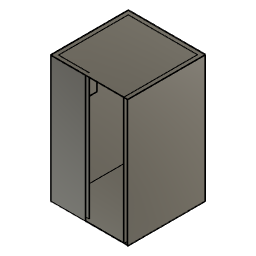
photo-booth v3 (Autodesk Fusion 360 design; units mm, degrees)
Autodesk Fusion 360 part; units mm, degrees
note: some values were not read from the file. Set by a fixed rule: which face or edge a step refers to.
sketch "Sketch1" plane through (0, 0, 0) normal (0, 0, 1) x (1, 0, 0)
  line L0 (0, 0) -> (1200, 0)
  line L1 (1200, 0) -> (1200, 1210)
  line L2 (1200, 1210) -> (0, 1210)
  line L3 (0, 1210) -> (0, 0)
  dimension "d1" = 1200
  dimension "d2" = 1210
  constraint horizontal L0
  constraint vertical L1
  constraint horizontal L2
  constraint vertical L3
  constraint coincident L0.start L3.end
  measures "d1" distance of L0.start L0.end
  measures "d2" distance of L0.start L2.end
extrude "Extrude1" add sketch "Sketch1" along normal blind 9 makes body 1 in component "Component"
sketch "Sketch2" plane through (1200, 0, 0) normal (1, 0, 0) x (0, 1, 0)
  line L0 (0, 0) -> (1210, 0)
  line L1 (1210, 0) -> (1210, 9)
  line L2 (1210, 9) -> (0, 9)
  line L3 (0, 9) -> (0, 0)
  line L4 (-9, 0) -> (1209, 0)
  line L5 (1209, 0) -> (1209, 2000)
  line L6 (1209, 2000) -> (-9, 2000)
  line L7 (-9, 2000) -> (-9, 0)
  dimension "d5" = 1218
  dimension "d6" = 2000
  constraint horizontal L4
  constraint vertical L5
  constraint horizontal L6
  constraint vertical L7
  measures "d5" distance of L4.start L4.end
  measures "d6" distance of L4.start L6.end
extrude "Extrude2" add sketch "Sketch2" along normal blind 9 bodies 1 in component "Component"
sketch "Sketch3" plane through (0, 1210, 0) normal (0, 1, 0) x (-1, 0, 0)
  line L0 (-1209, 0) -> (0, 0)
  line L1 (0, 0) -> (0, 9)
  line L2 (0, 9) -> (-1209, 9)
  line L3 (-1209, 0) -> (10, 0)
  line L4 (10, 0) -> (10, 2000)
  line L5 (10, 2000) -> (-1209, 2000)
  line L6 (-1209, 2000) -> (-1209, 0)
  line L7 (-1209, 9) -> (-1209, 0)
  dimension "d9" = 1219
  dimension "d10" = 2000
  constraint horizontal L3
  constraint vertical L4
  constraint horizontal L5
  constraint vertical L6
  constraint coincident L0.start L3.start
  measures "d9" distance of L0.start L3.end
  measures "d10" distance of L0.start L5.end
extrude "Extrude3" add sketch "Sketch3" along normal blind 9 separate body makes body 2 in component "Component"
sketch "Sketch6" plane through (0, 0, 0) normal (-1, 0, 0) x (0, -1, 0)
  line L0 (-1210, 0) -> (0, 0)
  line L1 (0, 0) -> (0, 9)
  line L2 (0, 9) -> (-1210, 9)
  line L3 (-1210, 9) -> (-1210, 0)
  line L4 (-1210, 0) -> (8, 0)
  line L5 (8, 0) -> (8, 2000)
  line L6 (8, 2000) -> (-1210, 2000)
  line L7 (-1210, 2000) -> (-1210, 0)
  dimension "d19" = 1218
  dimension "d20" = 2000
  constraint horizontal L4
  constraint vertical L5
  constraint horizontal L6
  constraint vertical L7
  measures "d19" distance of L0.start L4.end
  measures "d20" distance of L0.start L6.end
extrude "Extrude1'" add sketch "Sketch6" along normal blind 9 separate body makes body 3 in component "Component'"
sketch "Sketch7" plane through (1200, 0, 0) normal (-1, 0, 0) x (0, -1, 0)
  line L0 (0, 9) -> (0, 0)
  line L1 (0, 0) -> (9, 0)
  line L2 (9, 0) -> (9, 2000)
  line L3 (9, 2000) -> (-1209, 2000)
  line L4 (-1209, 2000) -> (-1209, 9)
  line L5 (-1209, 9) -> (0, 9)
  line L6 (-1209, 9) -> (-1159, 9)
  line L7 (-1159, 9) -> (-1159, 2000)
  line L8 (-1159, 2000) -> (-1209, 2000)
  line L9 (-1209, 2000) -> (-1209, 9)
  dimension "d23" = 50
  constraint horizontal L6
  constraint vertical L7
  constraint horizontal L8
  constraint vertical L9
  constraint coincident L4.end L5.start
  measures "d23" distance of L4.end L6.end
extrude "Extrude1''" add sketch "Sketch7" along normal blind 50 separate body contours L3 L4 L5 L6 L7 L8 L9 makes body 4
sketch "Sketch8" plane through (0, 0, 9) normal (0, 0, 1) x (-1, 0, 0)
  line L0 (0, -1210) -> (0, 0)
  line L1 (0, 0) -> (-1200, 0)
  line L2 (-1200, 0) -> (-1200, -1209)
  line L3 (-1209, -1210) -> (0, -1210)
  line L4 (0, -1210) -> (-50, -1210)
  line L5 (-50, -1210) -> (-50, -1160)
  line L6 (-50, -1160) -> (0, -1160)
  line L7 (0, -1160) -> (0, -1210)
  line L8 (-1200, -1209) -> (-1209, -1209)
  line L9 (-1209, -1209) -> (-1209, -1210)
  constraint horizontal L4
  constraint vertical L5
  constraint horizontal L6
  constraint vertical L7
  constraint coincident L0.start L3.end
extrude "Extrude2'" add sketch "Sketch8" along normal blind 1991 separate body contours L0 L3 L4 L5 L6 L7 makes body 5
sketch "Sketch9" plane through (0, 0, 9) normal (0, 0, 1) x (-1, 0, 0)
  line L0 (0, -1210) -> (0, 0)
  line L1 (0, 0) -> (-1200, 0)
  line L2 (-1200, 0) -> (-1200, -1209)
  line L3 (-1209, -1210) -> (0, -1210)
  line L4 (0, 0) -> (-50, 0)
  line L5 (-50, 0) -> (-50, -50)
  line L6 (-50, -50) -> (0, -50)
  line L7 (0, -50) -> (0, 0)
  line L8 (-1200, -1209) -> (-1209, -1209)
  line L9 (-1209, -1209) -> (-1209, -1210)
  constraint horizontal L4
  constraint vertical L5
  constraint horizontal L6
  constraint vertical L7
  constraint coincident L0.end L1.start
extrude "Extrude3'" add sketch "Sketch9" along normal blind 1991 separate body contours L0 L1 L4 L5 L6 L7 makes body 6
sketch "Sketch10" plane through (0, 1160, 0) normal (0, -1, 0) x (1, 0, 0)
  line L0 (0, 9) -> (50, 9)
  line L1 (50, 9) -> (50, 2000)
  line L2 (50, 2000) -> (0, 2000)
  line L3 (0, 2000) -> (0, 9)
  line L4 (0, 9) -> (50, 9)
  line L5 (50, 9) -> (50, 59)
  line L6 (50, 59) -> (0, 59)
  line L7 (0, 59) -> (0, 9)
  dimension "d30" = 50
  constraint horizontal L4
  constraint vertical L5
  constraint horizontal L6
  constraint vertical L7
  constraint coincident L0.start L3.end
  measures "d30" distance of L0.start L6.end
extrude "Extrude4" add sketch "Sketch10" along normal blind 1100 separate body contours L0 L1 L3 L4 L5 L6 L7 makes body 7
sketch "Sketch11" plane through (0, 1160, 0) normal (0, -1, 0) x (1, 0, 0)
  line L0 (0, 9) -> (50, 9)
  line L1 (50, 9) -> (50, 2000)
  line L2 (50, 2000) -> (0, 2000)
  line L3 (0, 2000) -> (0, 9)
  line L4 (0, 2000) -> (50, 2000)
  line L5 (50, 2000) -> (50, 1950)
  line L6 (50, 1950) -> (0, 1950)
  line L7 (0, 1950) -> (0, 2000)
  constraint horizontal L4
  constraint vertical L5
  constraint horizontal L6
  constraint vertical L7
  constraint coincident L1 L5.end
  constraint coincident L2.end L3.start
extrude "Extrude5" add sketch "Sketch11" along normal blind 1100 separate body contours L1 L2 L3 L4 L5 L6 L7 makes body 8
sketch "Sketch12" plane through (0, 0, 0) normal (1, 0, 0) x (0, 1, 0)
  line L0 (1210, 0) -> (1210, 2000)
  line L1 (1210, 2000) -> (-8, 2000)
  line L2 (-8, 2000) -> (-8, 0)
  line L3 (-8, 0) -> (1210, 0)
  line L4 (708, -17) -> (708, 1123) construction
  line L5 (600.0031, 1126.4153) -> (50.0031, 1126.4153) construction
  line L6 (525, 975) -> (710, 975)
  line L7 (710, 975) -> (710, 1310)
  line L8 (710, 1310) -> (525, 1310)
  line L9 (525, 1310) -> (525, 975)
  line L10 (525, 2000) -> (475, 2000)
  line L11 (475, 2000) -> (475, 50)
  line L12 (475, 50) -> (525, 50)
  line L13 (525, 50) -> (525, 2000)
  line L14 (710, 60) -> (660, 60)
  line L15 (660, 60) -> (660, 1950.3478)
  line L16 (660, 1950.3478) -> (710, 1950.3478)
  line L17 (710, 1950.3478) -> (710, 60)
  line L18 (525, 1950.1089) -> (475, 1950.1089)
  dimension "d35" = 1140
  dimension "d36" = 550
  dimension "d37" = 50
  dimension "d38" = 50
  constraint perpendicular L3 L4
  constraint parallel L1 L5
  constraint horizontal L6
  constraint vertical L7
  constraint horizontal L8
  constraint vertical L9
  constraint horizontal L10
  constraint vertical L11
  constraint horizontal L12
  constraint vertical L13
  constraint coincident L1 L10.start
  constraint horizontal L14
  constraint vertical L15
  constraint horizontal L16
  constraint vertical L17
  constraint coincident L13 L18.start
  constraint coincident L11 L18.end
  constraint perpendicular L11 L18
  measures "d35" distance of L4.start L4.end
  measures "d36" distance of L5.start L5.end
  measures "d37" distance of L10.start L10.end
  measures "d38" distance of L14.start L14.end
extrude "Extrude6" add sketch "Sketch12" along normal blind 50 separate body contours L9 L11 L12 L13 L18 | L8 L15 L16 L17 | L6 L7 L8 L15 L17 | L6 L14 L15 L17 makes body 9 at (16.6667, 525, 683.3696) makes body 10 at (0, 676.6667, 1320.2319)
sketch "Sketch13" plane through (0, 0, 0) normal (1, 0, 0) x (0, 1, 0)
  line L0 (1210, 0) -> (1210, 2000)
  line L1 (1210, 2000) -> (-8, 2000)
  line L2 (-8, 2000) -> (-8, 0)
  line L3 (-8, 0) -> (1210, 0)
  line L4 (475, 59) -> (475, 1199) construction
  line L5 (475, 1199) -> (1150, 1199)
  line L6 (1150, 1199) -> (1150, 1149)
  line L7 (1150, 1149) -> (475, 1149)
  line L8 (475, 1149) -> (475, 1199)
  line L9 (475, 1149) -> (49.9193, 1149)
  line L10 (49.9193, 1149) -> (49.9193, 1199)
  line L11 (49.9193, 1199) -> (475, 1199)
  line L12 (475, 1199) -> (475, 1149)
  line L13 (620.2773, 1199) -> (620.2773, 1529) construction
  line L14 (620.2773, 1529) -> (1150.6885, 1529)
  line L15 (1150.6885, 1529) -> (1150.6885, 1579)
  line L16 (1150.6885, 1579) -> (620.2773, 1579)
  line L17 (620.2773, 1579) -> (620.2773, 1529)
  line L18 (620.2773, 1529) -> (50.1055, 1529)
  line L19 (50.1055, 1529) -> (50.1055, 1579)
  line L20 (50.1055, 1579) -> (620.2773, 1579)
  line L21 (620.2773, 1579) -> (620.2773, 1529)
  dimension "d41" = 1140
  dimension "d42" = 50
  dimension "d43" = 330
  dimension "d44" = 50
  constraint parallel L0 L4
  constraint horizontal L5
  constraint vertical L6
  constraint horizontal L7
  constraint vertical L8
  constraint horizontal L9
  constraint vertical L10
  constraint horizontal L11
  constraint vertical L12
  constraint coincident L5 L13.start
  constraint perpendicular L5 L13
  constraint horizontal L14
  constraint vertical L15
  constraint horizontal L16
  constraint vertical L17
  constraint horizontal L18
  constraint vertical L19
  constraint horizontal L20
  constraint vertical L21
  measures "d41" distance of L4.start L4.end
  measures "d42" distance of L4.end L7.end
  measures "d43" distance of L13.start L13.end
  measures "d44" distance of L13.end L16.end
extrude "Extrude7" add sketch "Sketch13" along normal blind 50 separate body contours L5 L6 L7 L8 L12 | L8 L9 L10 L11 L12 | L14 L15 L16 L17 L21 | L17 L18 L19 L20 L21 makes body 11 at (16.6667, 783.8275, 1579) makes body 12 at (16.6667, 416.6128, 1199)
sketch "Sketch14" plane through (1150, 0, 0) normal (-1, 0, 0) x (0, -1, 0)
  line L0 (-1209, 2000) -> (-1209, 9)
  line L1 (-1209, 9) -> (-1159, 9)
  line L2 (-1159, 9) -> (-1159, 2000)
  line L3 (-1159, 2000) -> (-1209, 2000)
  line L4 (-1209, 2000) -> (-1159, 2000)
  line L5 (-1159, 2000) -> (-1159, 1950)
  line L6 (-1159, 1950) -> (-1209, 1950)
  line L7 (-1209, 1950) -> (-1209, 2000)
  constraint horizontal L4
  constraint vertical L5
  constraint horizontal L6
  constraint vertical L7
  constraint coincident L2 L5.end
  constraint coincident L0.start L3.end
extrude "Extrude8" add sketch "Sketch14" along normal blind 1100 separate body contours L0 L2 L3 L4 L5 L6 L7 makes body 13
sketch "Sketch15" plane through (1150, 0, 0) normal (-1, 0, 0) x (0, -1, 0)
  line L0 (-1209, 2000) -> (-1209, 9)
  line L1 (-1209, 9) -> (-1159, 9)
  line L2 (-1159, 9) -> (-1159, 2000)
  line L3 (-1159, 2000) -> (-1209, 2000)
  line L4 (-1209, 9) -> (-1159, 9)
  line L5 (-1159, 9) -> (-1159, 59)
  line L6 (-1159, 59) -> (-1209, 59)
  line L7 (-1209, 59) -> (-1209, 9)
  dimension "d49" = 50
  constraint horizontal L4
  constraint vertical L5
  constraint horizontal L6
  constraint vertical L7
  constraint coincident L0.end L1.start
  measures "d49" distance of L0.end L6.end
extrude "Extrude9" add sketch "Sketch15" along normal blind 1100 separate body contours L0 L1 L2 L4 L5 L6 L7 makes body 14
sketch "Sketch17" plane through (0, 1210, 0) normal (0, -1, 0) x (1, 0, 0)
  line L0 (1209, 0) -> (1209, 2000)
  line L1 (1209, 2000) -> (-10, 2000)
  line L2 (-10, 2000) -> (-10, 0)
  line L3 (-10, 0) -> (1209, 0)
  line L4 (1150, 1950) -> (50, 59)
  line L5 (1150, 59) -> (50, 1950)
  line L6 (50, 59) -> (50, 83.5)
  line L7 (1150, 59) -> (1150, 83)
  line L8 (50, 1950) -> (50, 1926)
  line L9 (1150, 1950) -> (1150, 1926)
  line L10 (1150, 1950) -> (1106.2, 1950)
  line L11 (50, 1950) -> (93.8, 1950)
  line L12 (50, 59) -> (93.8, 59)
  line L13 (1150, 59) -> (1106.2, 59)
  line L14 (1106.2, 59) -> (50, 1926)
  line L15 (93.8, 1950) -> (1150, 83)
  line L16 (93.8, 59) -> (1150, 1926)
  line L17 (1106.2, 1950) -> (50, 83.5)
  dimension "d54" = 43.8
  dimension "d55" = 43.8
  dimension "d56" = 43.8
  dimension "d57" = 43.8
  constraint vertical L6
  constraint vertical L7
  constraint vertical L8
  constraint vertical L9
  constraint perpendicular L9 L10
  constraint perpendicular L8 L11
  constraint perpendicular L6 L12
  constraint perpendicular L7 L13
  measures "d54" distance of L4.start L10.end
  measures "d55" distance of L5.end L11.end
  measures "d56" distance of L4.end L12.end
  measures "d57" distance of L5.start L13.end
extrude "Extrude11" add sketch "Sketch17" along normal blind 50 separate body contours L4 L9 L15 L16 | L4 L10 L15 L17 | L4 L5 L15 L16 | L4 L5 L15 L17 | L4 L5 L14 L16 | L4 L5 L14 L17 | L5 L11 L15 L17 | L5 L7 L15 L16 | L4 L12 L14 L16 | L4 L6 L14 L17 | L5 L13 L14 L16 | L5 L8 L14 L17 makes body 15
sketch "Sketch18" plane through (0, 0, 9) normal (0, 0, 1) x (-1, 0, 0)
  line L0 (0, -1210) -> (0, 0)
  line L1 (0, 0) -> (-1200, 0)
  line L2 (-1200, 0) -> (-1200, -1209)
  line L3 (-1209, -1210) -> (0, -1210)
  line L4 (-1200, 0) -> (-1150, 0)
  line L5 (-1150, 0) -> (-1150, -50)
  line L6 (-1150, -50) -> (-1200, -50)
  line L7 (-1200, -50) -> (-1200, 0)
  line L8 (-1200, -1209) -> (-1209, -1209)
  line L9 (-1209, -1209) -> (-1209, -1210)
  constraint horizontal L4
  constraint vertical L5
  constraint horizontal L6
  constraint vertical L7
  constraint coincident L1.end L2.start
extrude "Extrude4'" add sketch "Sketch18" along normal blind 1991 separate body contours L1 L2 L4 L5 L6 L7 makes body 16 in component "Component"
sketch "Sketch19" plane through (0, 1159, 0) normal (0, -1, 0) x (1, 0, 0)
  line L0 (1200, 9) -> (1200, 2000)
  line L1 (1200, 2000) -> (1150, 2000)
  line L2 (1150, 2000) -> (1150, 9)
  line L3 (1150, 9) -> (1200, 9)
  line L4 (1150, 1950) -> (1200, 1950)
  line L5 (1200, 1950) -> (1200, 2000)
  line L6 (1200, 2000) -> (1150, 2000)
  line L7 (1150, 2000) -> (1150, 1950)
  constraint horizontal L4
  constraint vertical L5
  constraint horizontal L6
  constraint vertical L7
  constraint coincident L0.end L1.start
  constraint coincident L2 L4.start
extrude "Extrude12" add sketch "Sketch19" along normal blind 1100 separate body contours L0 L1 L2 L4 L5 L6 L7 makes body 17
sketch "Sketch20" plane through (0, 1159, 0) normal (0, -1, 0) x (1, 0, 0)
  line L0 (1200, 9) -> (1200, 2000)
  line L1 (1200, 2000) -> (1150, 2000)
  line L2 (1150, 2000) -> (1150, 9)
  line L3 (1150, 9) -> (1200, 9)
  line L4 (1150, 9) -> (1201.209, 9)
  line L5 (1201.209, 9) -> (1201.209, 59)
  line L6 (1201.209, 59) -> (1150, 59)
  line L7 (1150, 59) -> (1150, 9)
  dimension "d64" = 50
  constraint horizontal L4
  constraint vertical L5
  constraint horizontal L6
  constraint vertical L7
  constraint coincident L2.end L3.start
  measures "d64" distance of L2.end L6.end
extrude "Extrude13" add sketch "Sketch20" along normal blind 1100 separate body contours L0 L2 L3 L4 L6 L7 makes body 18
sketch "Sketch21" plane through (1200, 0, 0) normal (-1, 0, 0) x (0, -1, 0)
  line L0 (0, 9) -> (0, 0)
  line L1 (0, 0) -> (9, 0)
  line L2 (9, 0) -> (9, 2000)
  line L3 (9, 2000) -> (-1209, 2000)
  line L4 (-1209, 2000) -> (-1209, 9)
  line L5 (-1209, 9) -> (0, 9)
  line L6 (-1150, 59) -> (-1106.2, 59)
  line L7 (-1150, 59) -> (-1150, 83)
  line L8 (-1150, 1950) -> (-1150, 1926)
  line L9 (-1150, 1950) -> (-1106.2, 1950)
  line L10 (-50, 60) -> (-93.8, 60)
  line L11 (-50, 60) -> (-50, 84)
  line L12 (-50, 1950) -> (-50, 1926)
  line L13 (-50, 1950) -> (-93.8, 1950)
  line L14 (-93.8, 60) -> (-1150, 1926)
  line L15 (-1106.2, 1950) -> (-50, 84)
  line L16 (-1106.2, 59) -> (-50, 1926)
  line L17 (-93.8, 1950) -> (-1150, 83)
  dimension "d67" = 43.8
  dimension "d68" = 24
  dimension "d69" = 24
  dimension "d70" = 43.8
  dimension "d71" = 43.8
  dimension "d72" = 24
  dimension "d73" = 24
  dimension "d74" = 43.8
  constraint horizontal L6
  constraint perpendicular L6 L7
  constraint vertical L8
  constraint perpendicular L8 L9
  constraint horizontal L10
  constraint perpendicular L10 L11
  constraint perpendicular L3 L12
  constraint perpendicular L12 L13
  measures "d67" distance of L6.start L6.end
  measures "d68" distance of L6.start L7.end
  measures "d69" distance of L8.start L8.end
  measures "d70" distance of L8.start L9.end
  measures "d71" distance of L10.start L10.end
  measures "d72" distance of L10.start L11.end
  measures "d73" distance of L12.start L12.end
  measures "d74" distance of L12.start L13.end
extrude "Extrude14" add sketch "Sketch21" along normal blind 50 separate body contours L6 L7 L14 L16 L17 | L10 L11 L14 L15 L16 | L14 L15 L16 L17 | L8 L9 L14 L15 L17 | L12 L13 L15 L16 L17 makes body 19
sketch "Sketch22" plane through (0, 1159, 0) normal (0, -1, 0) x (1, 0, 0)
  line L0 (1150, 9) -> (1150, 59)
  line L1 (1150, 59) -> (50, 59)
  line L2 (50, 59) -> (50, 9)
  line L3 (50, 9) -> (1150, 9)
  line L4 (50, 9) -> (1150, 9)
  line L5 (1150, 9) -> (1150, 2000)
  line L6 (1150, 2000) -> (50, 2000)
  line L7 (50, 2000) -> (50, 9)
  constraint horizontal L4
  constraint vertical L5
  constraint horizontal L6
  constraint vertical L7
  constraint coincident L2.end L3.start
extrude "Extrude1'''" add sketch "Sketch22" along normal blind 9 separate body makes body 20 in component "Component''"
sketch "Sketch25" plane through (1150, 0, 0) normal (-1, 0, 0) x (0, -1, 0)
  line L0 (-1159, 2000) -> (-1159, 1950)
  line L1 (-1159, 1950) -> (-59, 1950)
  line L2 (-59, 1950) -> (-59, 2000)
  line L3 (-59, 2000) -> (-1159, 2000)
  line L4 (-1140.9995, 2000) -> (9.0005, 2000)
  line L5 (9.0005, 2000) -> (9.0005, 9)
  line L6 (9.0005, 9) -> (-1140.9995, 9)
  line L7 (-1140.9995, 9) -> (-1140.9995, 2000)
  dimension "d83" = 1150
  dimension "d84" = 1991
  constraint horizontal L4
  constraint vertical L5
  constraint horizontal L6
  constraint vertical L7
  constraint coincident L3 L4.start
  measures "d83" distance of L4.start L4.end
  measures "d84" distance of L4.start L6.end
extrude "Extrude17" add sketch "Sketch25" along normal blind 9 separate body contours L1 L2 L3 L4 L7 | L1 L2 L4 L5 L6 L7 makes body 21
extrude "Extrude18" add 1 faces at (400, 0, 6) along direction (0, -1, 0) blind 9 separate body on bodies 1 makes body 22
sketch "Sketch26" plane through (0, 0, 9) normal (0, 0, 1) x (-1, 0, 0)
  line L0 (-1200, 0) -> (0, 0)
  line L1 (0, 0) -> (0, 9)
  line L2 (0, 9) -> (-1200, 9)
  line L3 (-1200, 9) -> (-1200, 0)
  line L4 (-1150, 0) -> (-1200, 0)
  line L5 (-1200, 0) -> (-1200, 9)
  line L6 (-1200, 9) -> (-1150, 9)
  line L7 (-1150, 9) -> (-1150, 0)
  constraint horizontal L4
  constraint vertical L5
  constraint horizontal L6
  constraint vertical L7
  constraint coincident L2.end L3.start
  constraint coincident L0 L4.start
extrude "Extrude19" add sketch "Sketch26" along normal blind 1991 separate body contours L0 L2 L3 L4 L5 L6 L7 makes body 23
extrude "Extrude20" add 1 faces at (1183.3333, 59, 1966.6667) along direction (0, -1, 0) blind 9 separate body on bodies 17 makes body 24
extrude "Extrude21" add 2 faces at (1147, 1140.9995, 1966.6667) (1147, 1140.9995, 656) along direction (0, 1, 0) blind 9 separate body on bodies 21 makes body 25
extrude "Extrude22" add 1 faces at (16.6667, 60, 1983.3333) along direction (0, -1, 0) blind 10 separate body on bodies 8 makes body 26
extrude "Extrude23" add 1 faces at (16.6667, 60, 42.3333) along direction (0, -1, 0) blind 10 separate body on bodies 7 makes body 27
sketch "Sketch27" plane through (0, 0, 9) normal (0, 0, 1) x (-1, 0, 0)
  line L0 (-1200, 0) -> (0, 0)
  line L1 (0, 0) -> (0, 9)
  line L2 (0, 9) -> (-1200, 9)
  line L3 (-1200, 9) -> (-1200, 0)
  line L4 (-1141, 0) -> (-541, 0)
  line L5 (-541, 9) -> (-49.9385, 9)
  line L6 (-49.9385, 9) -> (-49.9385, -50)
  line L7 (-49.9385, -50) -> (-541, -50)
  line L8 (-541, -50) -> (-541, 9)
  dimension "d99" = 600
  dimension "d100" = 59
  constraint coincident L0 L4.start
  constraint horizontal L5
  constraint vertical L6
  constraint horizontal L7
  constraint vertical L8
  constraint coincident L2 L5.start
  measures "d99" distance of L4.start L4.end
  measures "d100" distance of L5.start L7.end
extrude "Extrude24" add sketch "Sketch27" along normal blind 50 separate body contours L0 L6 L7 L8 makes body 28
sketch "Sketch28" plane through (0, 0, 59) normal (0, 0, 1) x (-1, 0, 0)
  line L0 (-541, -50) -> (-49.9385, -50)
  line L1 (-49.9385, -50) -> (-49.9385, 0)
  line L2 (-49.9385, 0) -> (-541, 0)
  line L3 (-541, 0) -> (-541, -50)
  line L4 (-541, 0) -> (-491, 0)
  line L5 (-491, 0) -> (-491, -50)
  line L6 (-491, -50) -> (-541, -50)
  line L7 (-541, -50) -> (-541, 0)
  dimension "d103" = 50
  dimension "d104" = 50
  constraint horizontal L4
  constraint vertical L5
  constraint horizontal L6
  constraint vertical L7
  constraint coincident L2.end L3.start
  measures "d103" distance of L2.end L4.end
  measures "d104" distance of L2.end L0.start
extrude "Extrude25" add sketch "Sketch28" along normal blind 1941 separate body contours L0 L2 L3 L4 L5 L6 L7 makes body 29
sketch "Sketch29" plane through (50, 0, 0) normal (1, 0, 0) x (0, 1, 0)
  line L0 (0, 9) -> (50, 9)
  line L1 (50, 9) -> (50, 2000)
  line L2 (50, 2000) -> (0, 2000)
  line L3 (0, 2000) -> (0, 9)
  line L4 (50, 1950) -> (0, 1950)
  line L5 (0, 1950) -> (0, 2000)
  line L6 (0, 2000) -> (50, 2000)
  line L7 (50, 2000) -> (50, 1950)
  constraint horizontal L4
  constraint vertical L5
  constraint horizontal L6
  constraint vertical L7
  constraint coincident L2.end L3.start
  constraint coincident L1 L4.start
extrude "Extrude26" add sketch "Sketch29" along normal blind 441 separate body contours L1 L2 L3 L4 L5 L6 L7 makes body 30
sketch "Sketch30" plane through (0, 0, 0) normal (0, -1, 0) x (1, 0, 0)
  line L0 (0, 9) -> (50, 9)
  line L1 (50, 9) -> (50, 2000)
  line L2 (50, 2000) -> (0, 2000)
  line L3 (0, 2000) -> (0, 9)
  line L4 (0, 2000) -> (540, 2000)
  line L5 (540, 2000) -> (540, 10)
  line L6 (540, 10) -> (0, 10)
  line L7 (0, 10) -> (0, 2000)
  constraint horizontal L4
  constraint vertical L5
  constraint horizontal L6
  constraint vertical L7
  constraint coincident L2.end L3.start
extrude "Extrude27" add sketch "Sketch30" along normal blind 9 separate body contours L1 L2 L3 L4 L6 L7 | L1 L4 L5 L6 makes body 31
sketch "Sketch31" plane through (0, 50, 0) normal (0, 1, 0) x (-1, 0, 0)
  line L0 (-50, 1950) -> (-50, 2000)
  line L1 (-50, 2000) -> (-491, 2000)
  line L2 (-491, 2000) -> (-491, 1950)
  line L3 (-491, 1950) -> (-50, 1950)
  line L4 (-50, 2000) -> (-540, 2000)
  line L5 (-540, 2000) -> (-540, 10)
  line L6 (-540, 10) -> (-50, 10)
  line L7 (-50, 10) -> (-50, 2000)
  constraint horizontal L4
  constraint vertical L5
  constraint horizontal L6
  constraint vertical L7
  constraint coincident L0.end L1.start
extrude "Extrude28" add sketch "Sketch31" along normal blind 9 separate body makes body 32
sketch "Sketch32" plane through (50, 0, 0) normal (1, 0, 0) x (0, 1, 0)
  line L0 (1160, 1950) -> (1160, 2000)
  line L1 (1160, 2000) -> (60, 2000)
  line L2 (60, 2000) -> (60, 1950)
  line L3 (60, 1950) -> (1160, 1950)
  line L4 (525, 1200) -> (660, 1200)
  line L5 (660, 1200) -> (660, 1529)
  line L6 (660, 1529) -> (525, 1529)
  line L7 (525, 1529) -> (525, 1200)
  line L8 (59, 2000) -> (1150, 2000)
  line L9 (1150, 2000) -> (1150, 9)
  line L10 (1150, 9) -> (59, 9)
  line L11 (59, 9) -> (59, 2000)
  constraint horizontal L4
  constraint vertical L5
  constraint horizontal L6
  constraint vertical L7
  constraint horizontal L8
  constraint vertical L9
  constraint horizontal L10
  constraint vertical L11
extrude "Extrude29" add sketch "Sketch32" along normal blind 9 separate body contours L2 L3 L8 L9 L10 L11 | L1 L2 L3 L8 L9 makes body 33
sketch "Sketch33" plane through (0, 0, 2000) normal (0, 0, 1) x (-1, 0, 0)
  line L0 (-50, -1160) -> (0, -1160)
  line L1 (0, -1160) -> (0, -60)
  line L2 (0, -60) -> (-50, -60)
  line L3 (-50, -60) -> (-50, -1160)
  line L4 (-1209, 9) -> (9, 9)
  line L5 (9, 9) -> (9, -1219)
  line L6 (9, -1219) -> (-1209, -1219)
  line L7 (-1209, -1219) -> (-1209, 9)
  constraint horizontal L4
  constraint vertical L5
  constraint horizontal L6
  constraint vertical L7
extrude "Extrude30" add sketch "Sketch33" along normal blind 9 separate body contours L0 L1 L2 L3 | L4 L5 L6 L7 makes body 34
component "Component" placed x (1, 0, 0) y (0, 1, 0) z (0, 0, 1) at (0, 0, 0)
component "Component'" placed x (1, 0, 0) y (0, 1, 0) z (0, 0, 1) at (0, 0, 0)
component "Component''" placed x (1, 0, 0) y (0, 1, 0) z (0, 0, 1) at (0, 0, 0)
hidden bodies 16
